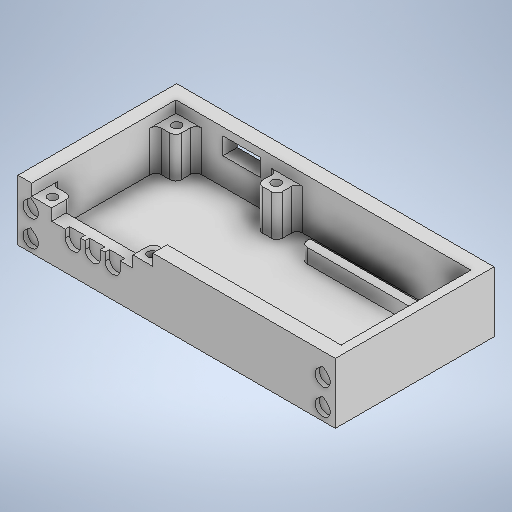
# Autodesk Inventor part: PowerModuleHousing
Saved by Autodesk Inventor 2025.1 (Build 291241020, 241B)
## iProperties
Created: 2024-09-25
Part Number: PowerModuleHousing
Material: Generic
Document SubType Name: Modeling
Designer: Si Teng Wu
Density: 1 g/cm^3
Appearance: Default
Author: Si Teng Wu
Autodesk Inventor part; units mm, degrees
ref_plane "YZ Plane" through (0, 0, 0) normal (1, 0, 0) x (0, 1, 0)
ref_plane "XZ Plane" through (0, 0, 0) normal (0, 1, 0) x (-1, 0, 0)
ref_plane "XY Plane" through (0, 0, 0) normal (0, 0, 1) x (1, 0, 0)
sketch "Sketch1" plane through (0, 0, 0) normal (0, 1, 0) x (-1, 0, 0)
  line L0 (55, 27.5) -> (-55, 27.5)
  line L1 (-55, 27.5) -> (-55, -27.5)
  line L2 (-55, -27.5) -> (55, -27.5)
  line L3 (55, -27.5) -> (55, 27.5)
  point P0 (0, 0)
  point P1 (-55, 0)
  point P2 (55, 0)
  dimension "d0" = 55
  dimension "d66" = 27.5
  dimension "d67" = 55
  dimension "d68" = 55
  constraints: 8 end point, 2 midpoint, 2 parallel, 1 horizontal, 1 perpendicular
  measures "d0" distance between parallel lines of L2 L0
  measures "d66" distance from line of L2 point (0, 0)
  measures "d67" distance of point (-55, 0) point (0, 0)
  measures "d68" distance of point (55, 0) point (0, 0)
extrude "Extrusion1" add sketch "Sketch1" along normal blind 21
sketch "Sketch2" plane through (0, 21, 0) normal (0, 1, 0) x (1, 0, 0)
  line L0 (-55, -27.5) -> (55, -27.5) projected
  line L1 (55, 27.5) -> (-55, 27.5) projected
  line L2 (52, -27.5) -> (-50.25, -27.5)
  line L3 (-50.25, -27.5) -> (-50.25, 27.5)
  line L4 (-50.25, 27.5) -> (52, 27.5)
  line L5 (52, 27.5) -> (52, -27.5)
  line L6 (-55, 27.5) -> (-55, -27.5) projected
  line L7 (55, -27.5) -> (55, 27.5) projected
  line L8 (-50.25, 27.5) -> (52, 27.5)
  line L9 (52, 27.5) -> (52, 22.5)
  line L10 (52, 22.5) -> (-50.25, 22.5)
  line L11 (-50.25, 22.5) -> (-50.25, 27.5)
  point P0 (0, 0)
  point P1 (52, 27.5)
  point P2 (-50.25, -27.5)
  point P3 (-50.25, 22.5)
  dimension "d122" = 50.25
  dimension "d333" = 5
  dimension "d338" = 52
  dimension "d354" = 102.25
  constraints: 16 end point, 4 parallel, 3 point on line, 2 horizontal, 2 perpendicular
  measures "d122" distance from line of L3 point (0, 0)
  measures "d333" distance between parallel lines of L1 L10
  measures "d338" distance from line of point (0, 0) L5
  measures "d354" distance between parallel lines of L5 L3
extrude "Extrusion2" cut sketch "Sketch2" against normal blind 18 contours L3 L10 L5 L0
sketch "Sketch11" plane through (0, 3, 0) normal (0, 1, 0) x (1, 0, 0)
  circle A0 centre (-12, 19) radius 1.55
  circle A1 centre (-12, -24) radius 1.55
  circle A2 centre (-46.5, 19) radius 1.55
  line L0 (-50.25, -27.5) -> (-50.25, 22.5) projected
  circle A3 centre (-46.5, -24) radius 1.55
  line L1 (52, -27.5) -> (-50.25, -27.5) projected
  line L2 (-50.25, 22.5) -> (52, 22.5) projected
  line L3 (-43.35, 22.5) -> (-50.25, 22.5)
  line L4 (-50.25, 22.5) -> (-50.25, 15.5)
  line L5 (-50.25, 15.5) -> (-43.35, 15.5)
  line L6 (-43.35, 15.5) -> (-43.35, 22.5)
  line L7 (-50.25, -20.5) -> (-43.35, -20.5)
  line L8 (-43.35, -20.5) -> (-43.35, -27.5)
  line L9 (-43.35, -27.5) -> (-50.25, -27.5)
  line L10 (-50.25, -27.5) -> (-50.25, -20.5)
  line L11 (-8.25, -27.5) -> (-15.15, -27.5)
  line L12 (-15.15, -27.5) -> (-15.15, -20.5)
  line L13 (-15.15, -20.5) -> (-8.25, -20.5)
  line L14 (-8.25, -20.5) -> (-8.25, -27.5)
  line L15 (-8.25, 22.5) -> (-15.15, 22.5)
  line L16 (-15.15, 22.5) -> (-15.15, 15.5)
  line L17 (-15.15, 15.5) -> (-8.25, 15.5)
  line L18 (-8.25, 15.5) -> (-8.25, 22.5)
  point P0 (-15.15, 22.5)
  dimension "d340" = 34.5
  dimension "d419" = 3.1
  dimension "d423" = 3.75
  dimension "d424" = 43
  dimension "d425" = 3.5
  dimension "d430" = 6.9
  dimension "d431" = 7
  dimension "d432" = 3.75
  constraints: 32 end point, 8 parallel, 6 point on line, 5 collinear, 4 centre point, 4 horizontal, 4 perpendicular, 3 equal radius, 2 equal length, 2 horizontal alignment, 2 vertical alignment
  measures "d340" distance of A0.centre A2.centre
  measures "d419" diameter of A0
  measures "d423" distance from line of L0 A2.centre
  measures "d424" distance of A3.centre A2.centre
  measures "d425" distance from line of L2 A2.centre
  measures "d430" distance of L4.end L5.end
  measures "d431" distance of L5.end L3.start
  measures "d432" distance from line of A0.centre L18
extrude "Extrusion17" add sketch "Sketch11" along normal blind 14
sketch "Sketch20" plane through (0, 3, 0) normal (0, 1, 0) x (1, 0, 0)
  line L0 (-50.25, -20.5) -> (-50.25, 22.5) projected
  line L1 (-8.25, -27.5) -> (-8.25, -20.5) projected
  line L2 (-8.25, -22.5) -> (52, -22.5)
  line L3 (52, -27.5) -> (-8.25, -27.5) projected
  line L4 (52, 22.5) -> (52, -27.5) projected
  point P0 (0, 0)
  point P1 (-50.25, -22.5)
  dimension "d439" = 5
  constraints: 3 point on line, 2 end point, 1 horizontal
  measures "d439" distance between parallel lines of L3 L2
extrude "Extrusion25" add sketch "Sketch20" along normal up to surface (18 mm away)
sketch "Sketch21" plane through (0, 3, 0) normal (0, 1, 0) x (1, 0, 0)
  line L0 (-43.35, -22.5) -> (-15.15, -22.5)
  line L1 (-15.15, -27.5) -> (-43.35, -27.5) projected
  line L2 (-43.35, -27.5) -> (-43.35, -20.5) projected
  line L3 (-15.15, -20.5) -> (-15.15, -27.5) projected
  point P0 (0, 0)
  dimension "d440" = 5
  constraints: 2 end point, 2 point on line, 1 horizontal, 1 perpendicular
  measures "d440" distance between parallel lines of L1 L0
extrude "Extrusion19" add sketch "Sketch21" along normal blind 10
fillet "Fillet7" radius 2 12 edges at (-8.25, 10, -15.5) (-15.15, 10, -15.5) (-15.15, 10, 20.5) (-8.25, 10, 20.5) (-43.35, 10, 20.5) (-43.35, 10, -15.5) (-43.35, 10, -22.5) (-50.25, 10, -15.5) (-15.15, 10, -22.5) (-50.25, 10, 20.5) (-8.25, 10, -22.5) (-8.25, 10, 22.5)
sketch "Sketch23" plane through (0, 3, 0) normal (0, 1, 0) x (1, 0, 0)
  line L0 (1.75, 17) -> (42, 17)
  line L1 (42, 17) -> (42, 14)
  line L2 (42, 14) -> (1.75, 14)
  line L3 (1.75, 14) -> (1.75, 17)
  line L4 (42, -14) -> (1.75, -14)
  line L5 (1.75, -14) -> (1.75, -17)
  line L6 (1.75, -17) -> (42, -17)
  line L7 (42, -17) -> (42, -14)
  line L8 (-50.25, -27.5) -> (-50.25, 22.5) projected
  line L9 (-50.25, 22.5) -> (52, 22.5) projected
  line L10 (52, 22.5) -> (52, -22.5) projected
  line L11 (-8.25, 17.5) -> (-8.25, 20.5) projected
  line L12 (0, 0) -> (40.25, 0)
  point P0 (21.875, -14)
  point P1 (21.875, 14)
  point P2 (-52, -22.5)
  point P3 (1.75, 15.5)
  point P4 (42, 15.5)
  point P5 (21.875, -17)
  point P6 (50.25, -27.5)
  point P7 (-10.3, 15.5)
  point P8 (-8.55, 22.5)
  dimension "d375" = 3
  dimension "d380" = 3
  dimension "d433" = 10
  dimension "d434" = 10
  dimension "d438" = 28
  constraints: 18 end point, 5 midpoint, 4 parallel, 3 horizontal, 2 collinear, 2 perpendicular, 4 other
  measures "d375" distance between parallel lines of L0 L2
  measures "d380" distance from line of L4 point (21.875, -17)
  measures "d438" distance between parallel lines of L4 L2
extrude "Extrusion21" add sketch "Sketch23" along normal blind 5
fillet "Fillet8" radius 2 4 edges at (1.75, 5.5, -14) (42, 5.5, -14) (42, 5.5, 14) (1.75, 5.5, 14)
chamfer "Chamfer33" distance 2 angle 45 2 edges at (21.875, 3, 17) (21.875, 3, -17)
sketch "Sketch25" plane through (55, 0, -27.5) normal (0, 0, -1) x (-1, 0, 0)
  line L0 (76, 18.33) -> (89, 18.33)
  line L1 (89, 18.33) -> (89, 12.33)
  line L2 (89, 12.33) -> (76, 12.33)
  line L3 (76, 12.33) -> (76, 18.33)
  line L4 (110, 0) -> (110, 21) projected
  line L5 (0, 21) -> (110, 21) projected
  dimension "d411" = 6
  dimension "d412" = 13
  dimension "d447" = 21
  dimension "d448" = 2.67
  constraints: 8 end point, 2 parallel, 1 horizontal, 1 perpendicular
  measures "d411" distance between parallel lines of L2 L0
  measures "d412" distance between parallel lines of L3 L1
  measures "d447" distance between parallel lines of L4 L1
  measures "d448" distance between parallel lines of L5 L0
extrude "Extrusion23" cut sketch "Sketch25" against normal up to surface (5 mm away)
sketch "Sketch24" plane through (-55, 0, 27.5) normal (0, 0, 1) x (1, 0, 0)
  circle A0 centre (105.6, 13) radius 2.65
  circle A1 centre (4.4, 13) radius 2.65
  circle A2 centre (105.6, 4) radius 2.65
  circle A3 centre (4.4, 4) radius 2.65
  line L0 (2.6689, 15.0064) -> (4.4, 16.5)
  line L1 (4.4, 16.5) -> (6.1311, 15.0064)
  line L2 (2.6689, 6.0064) -> (4.4, 7.5)
  line L3 (4.4, 7.5) -> (6.1311, 6.0064)
  line L4 (103.8689, 6.0064) -> (105.6, 7.5)
  line L5 (105.6, 7.5) -> (107.3311, 6.0064)
  line L6 (103.8689, 15.0064) -> (105.6, 16.5)
  line L7 (105.6, 16.5) -> (107.3311, 15.0064)
  line L8 (0, 0) -> (110, 0) projected
  line L9 (0, 0) -> (0, 21) projected
  line L10 (110, 0) -> (110, 21) projected
  circle A4 centre (19.05, 10.35) radius 2.65
  circle A5 centre (25.95, 10.35) radius 2.65
  circle A6 centre (32.85, 10.35) radius 2.65
  line L11 (11.65, 13) -> (39.85, 13) projected
  line L12 (16.4, 10.35) -> (16.4, 13)
  line L13 (21.7, 10.35) -> (21.7, 13)
  line L14 (23.3, 10.35) -> (23.3, 13)
  line L15 (28.6, 10.35) -> (28.6, 13)
  line L16 (30.2, 10.35) -> (30.2, 13)
  line L17 (35.5, 10.35) -> (35.5, 13)
  line L18 (4.75, 17) -> (11.65, 17) projected
  point P0 (55, 0)
  point P1 (20.0625, -1.6972)
  point P2 (19.05, 13)
  dimension "d391" = 5.3
  dimension "d399" = 3.5
  dimension "d409" = 4.4
  dimension "d410" = 4.4
  dimension "d450" = 6.9
  dimension "d451" = 6.9
  dimension "d452" = 2.65
  dimension "d453" = 4
  dimension "d454" = 19.05
  dimension "d455" = 9
  constraints: 28 end point, 14 point on circle, 14 tangent, 7 centre point, 6 equal radius, 6 perpendicular, 6 point on line, 5 horizontal alignment, 5 vertical alignment, 4 parallel
  measures "d391" diameter of A1
  measures "d399" distance of A1.centre L1.start
  measures "d409" distance from line of L9 A1.centre
  measures "d410" distance from line of L10 A0.centre
  measures "d450" distance of A5.centre A4.centre
  measures "d451" distance of A6.centre A5.centre
  measures "d452" distance from line of L11 A4.centre
  measures "d453" distance from line of L18 A1.centre
  measures "d454" distance from line of L9 A4.centre
  measures "d455" distance of A1.centre A3.centre
extrude "Extrusion22" cut sketch "Sketch24" against normal blind 1.55
sketch "Sketch28" plane through (0, 3, 0) normal (0, 1, 0) x (1, 0, 0)
  circle A0 centre (-46.5, 19) radius 1.55
  circle A1 centre (-12, 19) radius 1.55
  circle A2 centre (-12, -24) radius 1.55
  circle A3 centre (-46.5, -24) radius 1.55
  circle A4 centre (-46.5, -24) radius 1.55 projected
  circle A5 centre (-12, -24) radius 1.55 projected
  circle A6 centre (-12, 19) radius 1.55 projected
  circle A7 centre (-46.5, 19) radius 1.55 projected
  point P0 (0, 0)
  constraints: 8 concentric, 4 centre point
extrude "Extrusion26" add sketch "Sketch28" along normal blind 2
body "Solid1"
